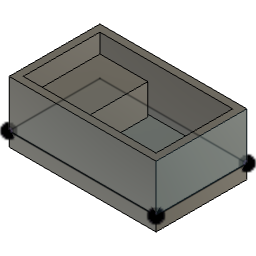
Goosebuster_case v2 (Autodesk Fusion 360 design; units mm, degrees)
Autodesk Fusion 360 part; units mm, degrees
note: some values were not read from the file. Set by a fixed rule: which sketch regions a step uses.
sketch "parts" plane through (0, 0, 0) normal (0, 0, 1) x (1, 0, 0)
  line L0 (-291.6, 172.4) -> (-190, 172.4)
  line L1 (-190, 172.4) -> (-190, 20)
  line L2 (-291.6, 20) -> (-291.6, 172.4)
  line L3 (-60, 106.2) -> (-20, 106.2)
  line L4 (-20, 106.2) -> (-20, 86.2)
  line L5 (-20, 86.2) -> (-60, 86.2)
  line L6 (-60, 86.2) -> (-60, 106.2)
  line L7 (-70, 172.4) -> (-20, 172.4)
  line L8 (-20, 172.4) -> (-20, 146.4)
  line L9 (-20, 146.4) -> (-70, 146.4)
  line L10 (-70, 146.4) -> (-70, 172.4)
  line L11 (-296.6, 177.4) -> (-15, 177.4)
  line L12 (-15, 177.4) -> (-15, 15)
  line L13 (-15, 15) -> (-296.6, 15)
  line L14 (-296.6, 15) -> (-296.6, 177.4)
  line L15 (-311.6, 192.4) -> (0, 192.4)
  line L16 (0, 192.4) -> (0, 0)
  line L17 (0, 0) -> (-311.6, 0)
  line L18 (-311.6, 0) -> (-311.6, 192.4)
  line L19 (-175, 20) -> (-141, 20)
  line L20 (-141, 20) -> (-141, 95)
  line L21 (-141, 95) -> (-175, 95)
  line L22 (-175, 95) -> (-175, 20)
  line L23 (-105, 75) -> (-20, 75)
  line L24 (-20, 75) -> (-20, 20)
  line L25 (-20, 20) -> (-105, 20)
  line L26 (-105, 20) -> (-105, 75)
  line L27 (-291.6, 20) -> (-190, 20)
  dimension "d75" = 152.4
  dimension "d76" = 101.6
  dimension "d77" = 34
  dimension "d78" = 75
  dimension "d79" = 55
  dimension "d80" = 85
  dimension "d81" = 40
  dimension "d82" = 20
  dimension "d83" = 26
  dimension "d84" = 50
  dimension "d85" = 281.6
  dimension "d86" = 162.4
  dimension "d87" = 192.4
  dimension "d88" = 311.6
  dimension "d89" = 5
  dimension "d90" = 5
  dimension "d91" = 5
  dimension "d92" = 15
  dimension "d93" = 5
  dimension "d94" = 5
  dimension "d95" = 5
  dimension "d96" = 5
  dimension "d97" = 71.2
  dimension "d98" = 15
  dimension "d99" = 15
  constraint horizontal L0
  constraint vertical L1
  constraint vertical L2
  constraint horizontal L3
  constraint vertical L4
  constraint horizontal L5
  constraint vertical L6
  constraint horizontal L7
  constraint vertical L8
  constraint horizontal L9
  constraint vertical L10
  constraint coincident L0.end L7
  constraint horizontal L11
  constraint vertical L12
  constraint horizontal L13
  constraint vertical L14
  constraint horizontal L15
  constraint vertical L16
  constraint horizontal L17
  constraint vertical L18
  constraint horizontal L19
  constraint vertical L20
  constraint horizontal L21
  constraint vertical L22
  constraint horizontal L23
  constraint vertical L24
  constraint horizontal L25
  constraint vertical L26
  constraint perpendicular L1 L27
  constraint coincident L16.end L17.start
  measures "d75" distance of L0.start L2.start
  measures "d76" distance of L0.start L0.end
  measures "d77" distance of L20.end L21.end
  measures "d78" distance of L19.end L20.end
  measures "d79" distance of L23.start L25.end
  measures "d80" distance of L23.start L23.end
  measures "d81" distance of L3.start L3.end
  measures "d82" distance of L3.start L5.end
  measures "d83" distance of L7.start L9.end
  measures "d84" distance of L7.start L7.end
  measures "d85" distance of L11.start L11.end
  measures "d86" distance of L11.end L12.end
  measures "d87" distance of L15.end L16.end
  measures "d88" distance of L15.start L15.end
  measures "d89" distance of L2 L14
  measures "d90" distance of L0 L11
  measures "d91" distance of L13 L19
  measures "d92" distance of L1 L22
  measures "d93" distance of L12 L24
  measures "d94" distance of L13 L25
  measures "d95" distance of L4 L12
  measures "d96" distance of L8 L12
  measures "d97" distance of L3 L11
  measures "d98" distance of L14 L18
  measures "d99" distance of L11 L15
extrude "Extrude5" add sketch "parts" along normal blind 65 contours L0 L1 L2 L27 makes body 1
extrude "Extrude6" add sketch "parts" along normal blind 19.9 separate body contours L19 L20 L21 L22 makes body 2
extrude "Extrude7" add sketch "parts" along normal blind 40.5 separate body contours L3 L4 L5 L6 makes body 3
extrude "Extrude8" add sketch "parts" along normal blind 18.5 separate body contours L7 L8 L9 L10 makes body 4
extrude "Extrude9" add sketch "parts" along normal blind 100 separate body contours L15 L16 L17 L18 makes body 5
sketch "base" plane through (0, 0, 0) normal (0, 0, 1) x (1, 0, 0)
  line L0 (-311.6, 0) -> (0, 0)
  line L1 (0, 0) -> (0, 192.4)
  line L2 (0, 192.4) -> (-311.6, 192.4)
  line L3 (-311.6, 192.4) -> (-311.6, 0)
  point P0 (-311.6, 0)
  point P1 (0, 192.4)
  constraint horizontal L0
  constraint vertical L1
  constraint horizontal L2
  constraint vertical L3
  constraint coincident P0 L0.start
  constraint coincident L0.end L1.start
  constraint coincident P1 L1.end
extrude "Extrude10" add sketch "base" against normal blind 30 separate body makes body 6
sketch "ports" plane through (0, 0, 0) normal (1, 0, 0) x (0, 1, 0)
  line L0 (0, 0) -> (192.4, 0)
  line L1 (192.4, 0) -> (192.4, 100)
  line L2 (192.4, 100) -> (0, 100)
  line L3 (0, 100) -> (0, 0)
extrude "Extrude11" add sketch "parts" along normal blind 15 separate body contours L23 L24 L25 L26 makes body 7
named bodies: "12V battery", "6V", "motor", "relay", "walls", "base", "rpi"
